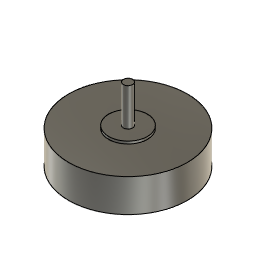
inwheel motor v2 (Autodesk Fusion 360 design; units mm, degrees)
Autodesk Fusion 360 part; units mm, degrees
sketch "スケッチ1" plane through (0, 0, 0) normal (0, 0, 1) x (1, 0, 0)
  circle A0 centre (0, 0) radius 83
  dimension "d1" = 166
  constraint coincident A0.centre origin
  measures "d1" diameter of A0
extrude "押し出し1" add sketch "スケッチ1" along normal blind 46
sketch "スケッチ2" plane through (0, 0, 46) normal (0, 0, 1) x (-1, 0, 0)
  circle A0 centre (0, 0) radius 83
  circle A1 centre (0, 0) radius 27.119
  constraint concentric A0 A1
extrude "押し出し2" add sketch "スケッチ2" along normal blind 3.5 contours A1
sketch "スケッチ3" plane through (0, 0, 49.5) normal (0, 0, 1) x (-1, 0, 0)
  circle A0 centre (0, 0) radius 27.119
  circle A1 centre (0, 0) radius 6.5
  dimension "d6" = 13
  constraint concentric A0 A1
  measures "d6" diameter of A1
extrude "押し出し3" add sketch "スケッチ3" along normal blind 52.5 contours A1
sketch "スケッチ4" plane through (0, 0, 0) normal (1, 0, 0) x (0, 1, 0)
  line L0 (6.5, 102) -> (-6.5, 102)
  line L1 (-6.5, 49.5) -> (6.5, 49.5)
  line L2 (6.5, 102) -> (6.5, 99)
  line L3 (6.5, 99) -> (3.5, 99)
  line L4 (3.5, 99) -> (3.5, 55)
  line L5 (3.5, 55) -> (6.5, 55)
  line L6 (6.5, 55) -> (6.5, 99)
  dimension "d9" = 3
  dimension "d10" = 44
  dimension "d11" = 3
  constraint coincident L0.start L2.start
  constraint perpendicular L0 L2
  constraint horizontal L3
  constraint vertical L4
  constraint horizontal L5
  constraint vertical L6
  measures "d9" distance of L0.start L2.end
  measures "d10" distance of L3 L5
  measures "d11" distance of L4 L6
extrude "押し出し4" cut sketch "スケッチ4" along normal blind 52.5 and the other way blind 60
sketch "スケッチ5" plane through (0, 0, 0) normal (0, 0, -1) x (1, 0, 0)
  circle A0 centre (0, 0) radius 83
  circle A1 centre (0, 0) radius 59.4788
  constraint coincident A0.centre A1.centre
extrude "押し出し5" add sketch "スケッチ5" along normal blind 9.5 contours A1
